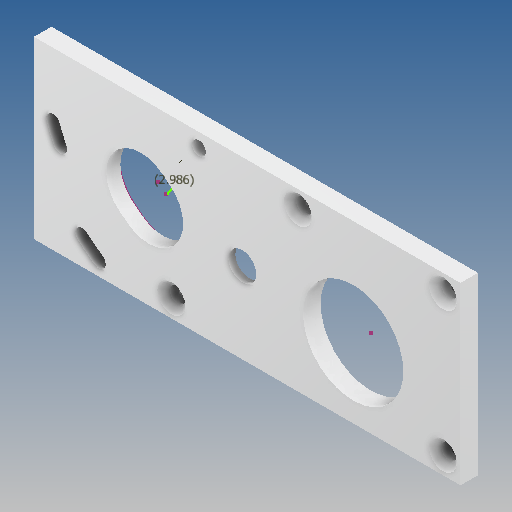
# Autodesk Inventor part: GEARBOX BACKPLATE
Saved by Autodesk Inventor 2020 (Build 240168000, 168)
## iProperties
Created: 2021-01-14
Part Number: GEARBOX BACKPLATE
Material: Aluminum 6061
Document SubType Name: Modeling
Designer: lucky
Density: 2.7 g/cm^3
Appearance: Aluminum - Flat
Mass: 62.5245 g
Surface Area: 130.779 cm^2
Volume: 23.1572 cm^3
Author: lucky
Revision Number: 5
Autodesk Inventor part; units mm, degrees
ref_plane "YZ Plane" through (0, 0, 0) normal (1, 0, 0) x (0, 1, 0)
ref_plane "XZ Plane" through (0, 0, 0) normal (0, 1, 0) x (-1, 0, 0)
ref_plane "XY Plane" through (0, 0, 0) normal (0, 0, 1) x (1, 0, 0)
sketch "MASTER SKETCH" plane through (0, 0, 0) normal (0, 0, 1) x (1, 0, 0)
  circle A0 centre (0, 0) radius 22.86
  circle A1 centre (-31.6504, 3.081) radius 8.89
  circle A2 centre (-31.6504, 3.081) radius 20.32
  circle A3 centre (-60.6627, 6.8802) radius 8.89
  circle A4 centre (-58.2971, 5.0584) radius 6.35
  circle A5 centre (-60.6627, 6.8802) radius 25.4
  circle A6 centre (-58.2971, 5.0584) radius 25.4 construction
  line L0 (-44.0087, 26.0584) -> (-77.3167, -12.298) construction
  line L1 (-68.9445, 30.8921) -> (-52.3809, -17.1317) construction
  circle A7 centre (-44.0087, 26.0584) radius 2
  arc A8 (-68.9445, 30.8921) -> (-69.3394, 27.9326) centre (-44.0087, 26.0584) ccw construction
  arc A9 (-70.9079, 31.2727) -> (-71.334, 28.0802) centre (-44.0087, 26.0584) ccw
  arc A10 (-66.981, 30.5115) -> (-67.3449, 27.785) centre (-44.0087, 26.0584) ccw
  arc A11 (-66.981, 30.5115) -> (-70.9079, 31.2727) centre (-68.9445, 30.8921) ccw
  arc A12 (-71.334, 28.0802) -> (-67.3449, 27.785) centre (-69.3394, 27.9326) ccw
  arc A13 (-85.5985, 11.7139) -> (-83.6279, 6.9326) centre (-44.0087, 26.0584) ccw construction
  arc A14 (-87.4892, 11.0618) -> (-85.429, 6.0631) centre (-44.0087, 26.0584) ccw
  arc A15 (-83.7078, 12.366) -> (-81.8268, 7.8021) centre (-44.0087, 26.0584) ccw
  arc A16 (-83.7078, 12.366) -> (-87.4892, 11.0618) centre (-85.5985, 11.7139) ccw
  arc A17 (-85.429, 6.0631) -> (-81.8268, 7.8021) centre (-83.6279, 6.9326) ccw
  arc A18 (-77.3167, -12.298) -> (-72.5856, -15.9416) centre (-44.0087, 26.0584) ccw construction
  arc A19 (-78.6281, -13.8081) -> (-73.7107, -17.5951) centre (-44.0087, 26.0584) ccw
  arc A20 (-76.0054, -10.7879) -> (-71.4605, -14.288) centre (-44.0087, 26.0584) ccw
  arc A21 (-76.0054, -10.7879) -> (-78.6281, -13.8081) centre (-77.3167, -12.298) ccw
  arc A22 (-73.7107, -17.5951) -> (-71.4605, -14.288) centre (-72.5856, -15.9416) ccw
  arc A23 (-52.3809, -17.1317) -> (-47.2548, -17.8157) centre (-44.0087, 26.0584) ccw construction
  arc A24 (-52.7615, -19.0951) -> (-47.4024, -19.8103) centre (-44.0087, 26.0584) ccw
  arc A25 (-52.0003, -15.1682) -> (-47.1072, -15.8212) centre (-44.0087, 26.0584) ccw
  arc A26 (-52.0003, -15.1682) -> (-52.7615, -19.0951) centre (-52.3809, -17.1317) ccw
  arc A27 (-47.4024, -19.8103) -> (-47.1072, -15.8212) centre (-47.2548, -17.8157) ccw
  arc A28 (-35.7269, 2.0465) -> (-32.9664, 3.1843) centre (-44.0087, 26.0584) ccw construction
  arc A29 (-35.0748, 0.1558) -> (-32.0969, 1.3831) centre (-44.0087, 26.0584) ccw
  arc A30 (-36.379, 3.9372) -> (-33.8358, 4.9854) centre (-44.0087, 26.0584) ccw
  arc A31 (-36.379, 3.9372) -> (-35.0748, 0.1558) centre (-35.7269, 2.0465) ccw
  arc A32 (-32.0969, 1.3831) -> (-33.8358, 4.9854) centre (-32.9664, 3.1843) ccw
  line L2 (-91.0627, 30.0584) -> (30.5868, 30.0584)
  line L3 (30.5868, 30.0584) -> (30.5868, -19.9416)
  line L4 (30.5868, -19.9416) -> (-91.0627, -19.9416)
  line L5 (-91.0627, -19.9416) -> (-91.0627, 30.0584)
  circle A33 centre (0, 0) radius 14.2875 construction
  circle A34 centre (25.5868, -14.9416) radius 3
  circle A35 centre (25.5868, 25.0584) radius 3
  circle A36 centre (-51.8755, -14.9416) radius 3
  line L6 (-91.0627, 25.3566) -> (30.5868, 25.3566) construction
  circle A37 centre (-15.8118, 25.0584) radius 3
  line L7 (-58.2971, 5.0584) -> (-60.6627, 6.8802) construction
  line L8 (-52.3328, 12.803) -> (-54.6984, 14.6248)
  line L9 (-66.627, -0.8643) -> (-64.2614, -2.6861)
  arc A38 (-64.2614, -2.6861) -> (-52.3328, 12.803) centre (-58.2971, 5.0584) ccw
  arc A39 (-54.6984, 14.6248) -> (-66.627, -0.8643) centre (-60.6627, 6.8802) ccw
  circle A40 centre (0, 0) radius 24.13 construction
  circle A41 centre (-31.6504, 3.081) radius 21.59 construction
  line L10 (-67.5422, -2.0527) -> (-65.1767, -3.8745)
  arc A42 (-65.1767, -3.8745) -> (-51.4176, 13.9914) centre (-58.2971, 5.0584) ccw
  line L11 (-51.4176, 13.9914) -> (-53.7832, 15.8132)
  arc A43 (-53.7832, 15.8132) -> (-67.5422, -2.0527) centre (-60.6627, 6.8802) ccw
  circle A44 centre (-44.0087, 26.0584) radius 50.8 construction
  arc A45 (-67.3815, -0.857) -> (-64.0616, -3.4137) centre (-44.0087, 26.0584) ccw
  arc A46 (-53.9439, 14.6174) -> (-52.5326, 13.5306) centre (-44.0087, 26.0584) ccw
  arc A47 (-53.9439, 14.6174) -> (-67.3815, -0.857) centre (-60.6627, 6.8802) ccw
  arc A48 (-64.0616, -3.4137) -> (-52.5326, 13.5306) centre (-58.2971, 5.0584) ccw
  line L12 (-35.7269, 2.0465) -> (-85.5985, 11.7139) construction
  point P0 (-60.0285, -7.7006)
  point P1 (-59.4799, 5.9693)
  dimension "d0" = 45.72
  dimension "d1" = 17.78
  dimension "d2" = 40.64
  dimension "d4" = 17.78
  dimension "d5" = 12.7
  dimension "d6" = 50.8
  dimension "d9" = 50.8
  dimension "d10" = 60
  dimension "d12" = 4
  dimension "d13" = 4
  dimension "d14" = 4
  dimension "d15" = 4
  dimension "d16" = 4
  dimension "d17" = 4
  dimension "d19" = 28.575
  dimension "d28" = 6
  dimension "d29" = 6
  dimension "d30" = 6
  dimension "d39" = 31.8
  dimension "d42" = 29.26
  dimension "d43" = 26.72
  dimension "d70" = 2
  dimension "d73" = 6
  dimension "d84" = 2
  dimension "d85" = 5
  dimension "d89" = 19.55
  dimension "d108" = 1.27
  dimension "d109" = 1.27
  dimension "d110" = 2.5
  dimension "d111" = 2.5
  dimension "d113" = 2.5
  dimension "d114" = 2
  dimension "d129" = 1.5
  dimension "d133" = 2.5
  dimension "d136" = 50
  dimension "d139" = 2
  dimension "d140" = 2.5
  dimension "d141" = 2
  dimension "d142" = 2
  dimension "d181" = 60
  constraints: 78 point on circle, 48 centre point, 28 end point, 28 tangent, 12 coincident, 6 midpoint, 4 parallel, 2 perpendicular, 2 point on line, 1 concentric, 1 horizontal, 1 horizontal alignment, 1 vertical alignment, 10 other
  measures "d0" diameter of A0
  measures "d1" diameter of A1
  measures "d2" diameter of A2
  measures "d4" diameter of A3
  measures "d5" diameter of A4
  measures "d6" diameter of A5
  measures "d9" diameter of A6
  measures "d10" angle of L1 L0
  measures "d12" diameter of A7
  measures "d13" diameter of A12
  measures "d14" diameter of A17
  measures "d15" diameter of A22
  measures "d16" diameter of A27
  measures "d17" diameter of A32
  measures "d19" diameter of A33
  measures "d28" diameter of A34
  measures "d29" diameter of A35
  measures "d30" diameter of A36
  measures "d39" distance of A0.centre A1.centre
  measures "d42" distance of A1.centre A3.centre
  measures "d43" distance of A1.centre A4.centre
  measures "d70" distance edge to line of A34 L4
  measures "d73" diameter of A37
  measures "d84" distance edge to line of A36 L4
  measures "d85" distance edge to line of A5 L5
  measures "d89" diameter of A39
  measures "d108" radial gap between concentric circles of A0 A40
  measures "d109" radial gap between concentric circles of A2 A41
  measures "d114" distance edge to line of A22 L4
  measures "d129" radial gap between concentric circles of A39 A43
  measures "d136" distance between parallel lines of L4 L2
  measures "d139" distance edge to line of A7 L2
  measures "d141" distance edge to line of A37 L2
  measures "d142" distance edge to line of A34 L3
  measures "d181" angle of L0 L12
sketch "Sketch2" plane through (0, 0, 0) normal (0, 0, 1) x (1, 0, 0)
  line L0 (-91.0627, 30.0584) -> (30.5868, 30.0584) projected
  line L1 (-91.0627, -19.9416) -> (-91.0627, 30.0584) projected
  line L2 (30.5868, 30.0584) -> (30.5868, -19.9416) projected
  line L3 (30.5868, -19.9416) -> (-91.0627, -19.9416) projected
  line L4 (-91.0627, 30.0584) -> (30.5868, 30.0584)
  line L5 (30.5868, 30.0584) -> (30.5868, -19.9416)
  line L6 (30.5868, -19.9416) -> (-91.0627, -19.9416)
  line L7 (-91.0627, -19.9416) -> (-91.0627, 30.0584)
  point P0 (0, 0)
  constraints: 8 end point, 2 parallel, 1 horizontal, 1 perpendicular
extrude "Extrusion1" add sketch "Sketch2" along normal blind 5
sketch "Sketch3" plane through (0, 0, 0) normal (0, 0, -1) x (-1, 0, 0)
  arc A0 (47.1072, -15.8212) -> (47.4024, -19.8103) centre (47.2548, -17.8157) ccw projected
  arc A1 (47.1072, -15.8212) -> (52.0003, -15.1682) centre (44.0087, 26.0584) ccw projected
  arc A2 (47.4024, -19.8103) -> (52.7615, -19.0951) centre (44.0087, 26.0584) ccw projected
  arc A3 (52.7615, -19.0951) -> (52.0003, -15.1682) centre (52.3809, -17.1317) ccw projected
  line L0 (91.0627, 30.0584) -> (91.0627, -19.9416) projected
  line L1 (-30.5868, 30.0584) -> (91.0627, 30.0584) projected
  line L2 (-30.5868, -19.9416) -> (-30.5868, 30.0584) projected
  line L3 (91.0627, -19.9416) -> (-30.5868, -19.9416) projected
  arc A4 (71.4605, -14.288) -> (73.7107, -17.5951) centre (72.5856, -15.9416) ccw projected
  arc A5 (73.7107, -17.5951) -> (78.6281, -13.8081) centre (44.0087, 26.0584) ccw projected
  arc A6 (71.4605, -14.288) -> (76.0054, -10.7879) centre (44.0087, 26.0584) ccw projected
  arc A7 (78.6281, -13.8081) -> (76.0054, -10.7879) centre (77.3167, -12.298) ccw projected
  arc A8 (81.8268, 7.8021) -> (83.7078, 12.366) centre (44.0087, 26.0584) ccw projected
  arc A9 (81.8268, 7.8021) -> (85.429, 6.0631) centre (83.6279, 6.9326) ccw projected
  arc A10 (85.429, 6.0631) -> (87.4892, 11.0618) centre (44.0087, 26.0584) ccw projected
  arc A11 (87.4892, 11.0618) -> (83.7078, 12.366) centre (85.5985, 11.7139) ccw projected
  arc A12 (71.334, 28.0802) -> (70.9079, 31.2727) centre (44.0087, 26.0584) ccw projected
  arc A13 (67.3449, 27.785) -> (66.981, 30.5115) centre (44.0087, 26.0584) ccw projected
  arc A14 (70.9079, 31.2727) -> (66.981, 30.5115) centre (68.9445, 30.8921) ccw projected
  arc A15 (67.3449, 27.785) -> (71.334, 28.0802) centre (69.3394, 27.9326) ccw projected
  arc A16 (66.627, -0.8643) -> (54.6984, 14.6248) centre (60.6627, 6.8802) ccw projected
  arc A17 (52.3328, 12.803) -> (64.2614, -2.6861) centre (58.2971, 5.0584) ccw projected
  line L4 (52.3328, 12.803) -> (54.6984, 14.6248) projected
  line L5 (66.627, -0.8643) -> (64.2614, -2.6861) projected
  point P0 (0, 0)
extrude "Extrusion2" cut sketch "Sketch3" against normal blind 5 contours A6 A7 A5 A4 | A8 A11 A10 A9 | L5 A17 L4 A16
sketch "Sketch4" plane through (0, 0, 0) normal (0, 0, -1) x (-1, 0, 0)
  circle A0 centre (-25.5868, 25.0584) radius 3 projected
  circle A1 centre (15.8118, 25.0584) radius 3 projected
  circle A2 centre (51.8755, -14.9416) radius 3 projected
  circle A3 centre (-25.5868, -14.9416) radius 3 projected
  point P0 (0, 0)
sketch "Sketch5" plane through (0, 0, 0) normal (0, 0, -1) x (-1, 0, 0)
  circle A0 centre (0, 0) radius 22.86 projected
hole "Hole1" at (0, 0, 0) direction (0, 0, 1) diameter 28.575 end through all
hole "Hole2" at (25.5868, 25.0584, 0) at (-15.8118, 25.0584, 0) at (25.5868, -14.9416, 0) at (-51.8755, -14.9416, 0) direction (0, 0, 1) diameter 4.5 end through all counterbore diameter 6 counterbore depth 1
sketch "Sketch6" plane through (0, 0, 0) normal (0, 0, -1) x (-1, 0, 0)
  line L0 (91.0627, 25.3566) -> (-30.5868, 25.3566) construction
  circle A0 centre (44.0087, 26.0584) radius 2 projected
  point P0 (0, 0)
hole "Hole3" at (-44.0087, 26.0584, 0) direction (0, 0, 1) diameter 4 end through all
sketch "Sketch7" plane through (0, 0, 0) normal (0, 0, -1) x (-1, 0, 0)
  circle A0 centre (31.6504, 3.081) radius 20.32 projected
  point P0 (0, 0)
hole "Hole4" at (-31.6504, 3.081, 0) direction (0, 0, 1) diameter 8 depth 5 counterbore diameter 22 counterbore depth 3
sketch "Sketch8" plane through (0, 0, 0) normal (0, 0, -1) x (-1, 0, 0)
  arc A0 (52.3328, 12.803) -> (64.2614, -2.6861) centre (58.2971, 5.0584) ccw projected
  line L0 (66.627, -0.8643) -> (64.2614, -2.6861) projected
  arc A1 (66.627, -0.8643) -> (54.6984, 14.6248) centre (60.6627, 6.8802) ccw projected
  line L1 (52.3328, 12.803) -> (54.6984, 14.6248) projected
  arc A2 (67.5422, -2.0527) -> (53.7832, 15.8132) centre (60.6627, 6.8802) ccw projected
  line L2 (51.4176, 13.9914) -> (53.7832, 15.8132) projected
  line L3 (67.5422, -2.0527) -> (65.1767, -3.8745) projected
  arc A3 (51.4176, 13.9914) -> (65.1767, -3.8745) centre (58.2971, 5.0584) ccw projected
  point P0 (0, 0)
extrude "Extrusion3" cut sketch "Sketch8" against normal blind 1 contours L1 A1 L0 A0 | L3 A3 L2 A2
sketch "Sketch11" plane through (0, 0, 0) normal (0, 0, 1) x (1, 0, 0)
  line L0 (30.5868, -19.9416) -> (30.5868, 30.0584) projected
  line L1 (30.5868, 30.0584) -> (30.5868, -19.9416)
  line L2 (30.5868, -19.9416) -> (-61.3292, -19.9416)
  line L3 (-91.0627, -19.9416) -> (30.5868, -19.9416) projected
  line L4 (-61.3292, -19.9416) -> (-32.4617, 30.0584)
  line L5 (30.5868, 30.0584) -> (-91.0627, 30.0584) projected
  line L6 (-32.4617, 30.0584) -> (30.5868, 30.0584)
  circle A0 centre (-44.0087, 26.0584) radius 2 projected
  point P0 (0, 0)
  dimension "d147" = 120
  dimension "d148" = 8
  constraints: 8 end point, 2 point on line, 1 collinear, 1 parallel
  measures "d147" angle of L4 L5
  measures "d148" distance from line of A0.centre L4
extrude "Extrusion5" [suppressed]
sketch "Sketch12" plane through (0, 0, 0) normal (0, 0, 1) x (1, 0, 0)
  circle A0 centre (-15.8118, 25.0584) radius 3 projected
  circle A1 centre (25.5868, 25.0584) radius 3 projected
  circle A2 centre (25.5868, -14.9416) radius 3 projected
  circle A3 centre (-51.8755, -14.9416) radius 3 projected
  point P0 (0, 0)
hole "Hole5" [suppressed]
sketch "Sketch13" plane through (0, 0, 0) normal (0, 0, 1) x (1, 0, 0)
  circle A0 centre (0, 0) radius 14.2875 construction
hole "Hole6" [suppressed]
sketch "Sketch14" plane through (0, 0, 0) normal (0, 0, 1) x (1, 0, 0)
  circle A0 centre (-31.6504, 3.081) radius 8.89 projected
  point P0 (0, 0)
hole "Hole7" [suppressed]
sketch "Sketch15" plane through (0, 0, 5) normal (0, 0, 1) x (1, 0, 0)
  circle A0 centre (-15.8118, 25.0584) radius 2.25 projected
  circle A1 centre (-51.8755, -14.9416) radius 2.25 projected
  circle A2 centre (25.5868, 25.0584) radius 2.25 projected
  circle A3 centre (25.5868, -14.9416) radius 2.25 projected
  point P0 (0, 0)
hole "Hole8" at (-15.8118, 25.0584, 5) at (-51.8755, -14.9416, 5) at (25.5868, -14.9416, 5) at (25.5868, 25.0584, 5) direction (0, 0, -1) diameter 4 end through all countersink diameter 8 countersink angle 90
sketch "Sketch16" plane through (0, 0, 0) normal (0, 0, -1) x (-1, 0, 0)
  circle A0 centre (44.0087, 26.0584) radius 2 projected
  arc A1 (67.5422, -2.0527) -> (53.7832, 15.8132) centre (60.6627, 6.8802) ccw projected
  line L0 (51.4176, 13.9914) -> (53.7832, 15.8132) projected
  arc A2 (51.4176, 13.9914) -> (65.1767, -3.8745) centre (58.2971, 5.0584) ccw projected
  line L1 (67.5422, -2.0527) -> (65.1767, -3.8745) projected
  arc A3 (71.4605, -14.288) -> (76.0054, -10.7879) centre (44.0087, 26.0584) ccw projected
  arc A4 (78.6281, -13.8081) -> (76.0054, -10.7879) centre (77.3167, -12.298) ccw projected
  arc A5 (73.7107, -17.5951) -> (78.6281, -13.8081) centre (44.0087, 26.0584) ccw projected
  arc A6 (71.4605, -14.288) -> (73.7107, -17.5951) centre (72.5856, -15.9416) ccw projected
  line L2 (58.1824, 5.2073) -> (44.0087, 26.0584)
  point P0 (0, 0)
  dimension "d180" = 2.9858
  constraints: 2 end point
  measures "d180" distance of L0.start L0.end
equation "\"d0\" = SR2PD"
equation "\"d1\" = SR1PD"
equation "\"d2\" = FirstReductionPD"
equation "\"d4\" = Pinion4inPD"
equation "\"d5\" = PinionPD"
equation "\"PinionPD\" = 12.7"
equation "\"FirstReductionPD\" = 40.64"
equation "\"HighGearPD\" = 20.32"
equation "\"LowGearPD\" = 17.78"
equation "\"HighGearDogPD\" = 63.5"
equation "\"LowGearDogPD\" = 76.2"
equation "\"SR1PD\" = 17.78"
equation "\"SR2PD\" = 45.72"
equation "\"Pinion4inPD\" = 17.78"
body "Solid1"
